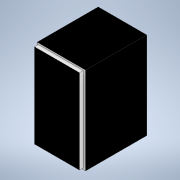
# Autodesk Inventor part: battery
Saved by Autodesk Inventor 2022 (Build 260153000, 153)
## iProperties
Created: 2022-08-22
Part Number: battery
Material: LCP Plastic
Document SubType Name: Modeling
Designer: Sachin
Density: 1.626 g/cm^3
Appearance: Smooth - White
Author: Sachin
Autodesk Inventor part; units mm, degrees
ref_plane "YZ Plane" through (0, 0, 0) normal (1, 0, 0) x (0, 1, 0)
ref_plane "XZ Plane" through (0, 0, 0) normal (0, 1, 0) x (-1, 0, 0)
ref_plane "XY Plane" through (0, 0, 0) normal (0, 0, 1) x (1, 0, 0)
sketch "Sketch1" plane through (0, 0, 0) normal (0, 0, 1) x (1, 0, 0)
  line L0 (0, 0) -> (-63.5, 0)
  line L1 (-63.5, 0) -> (-63.5, 114.3)
  line L2 (-63.5, 114.3) -> (0, 114.3)
  line L3 (0, 114.3) -> (0, 0)
  dimension "d0" = 63.5
  dimension "d1" = 114.3
  constraints: 8 end point, 2 parallel, 1 horizontal, 1 perpendicular
  measures "d0" distance of L1.end L2.end
  measures "d1" distance of L0.end L1.end
extrude "Extrusion1" add sketch "Sketch1" along normal blind 85
sketch "Sketch2" plane through (0, 0, 85) normal (0, 0, 1) x (1, 0, 0)
  line L0 (0, 114.3) -> (-63.5, 114.3) projected
  line L1 (-63.5, 114.3) -> (-63.5, 0) projected
  line L2 (0, 114.3) -> (-63.5, 114.3)
  line L3 (-63.5, 114.3) -> (-63.5, 0)
  line L4 (-63.5, 0) -> (0, 0)
  line L5 (0, 0) -> (0, 114.3)
  point P0 (0, 0)
  constraints: 8 end point, 2 parallel, 1 horizontal, 1 perpendicular
extrude "Extrusion2" cut sketch "Sketch2" against normal blind 5
sketch "Sketch3" plane through (0, 0, 80) normal (0, 0, 1) x (1, 0, 0)
  line L0 (-3.0089, 112.3665) -> (-61.8666, 112.3665)
  line L1 (-61.8666, 112.3665) -> (-61.8666, 1.9046)
  line L2 (-61.8666, 1.9046) -> (-3.0089, 1.9046)
  line L3 (-3.0089, 1.9046) -> (-3.0089, 112.3665)
  point P0 (0, 0)
  constraints: 8 end point, 2 parallel, 1 horizontal, 1 perpendicular
extrude "Extrusion3" add sketch "Sketch3" along normal blind 5
body "Solid1"
